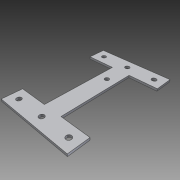
# Autodesk Inventor part: Shooter I Brace
Saved by Autodesk Inventor 2014 SP1 (Build 180222100, 222)
## iProperties
Created: 2013-12-15
Part Number: Shooter I Brace
Material: Aluminum 6061
Document SubType Name: Modeling
Designer: Moses
Mass: 64.49 g
Surface Area: 175.547 cm^2
Volume: 23.7971 cm^3
Density: 2.71 g/cm^3
Appearance: Aluminum - Flat
Author: Moses
Autodesk Inventor part; units mm, degrees
ref_plane "YZ Plane" through (0, 0, 0) normal (1, 0, 0) x (0, 1, 0)
ref_plane "XZ Plane" through (0, 0, 0) normal (0, 1, 0) x (-1, 0, 0)
ref_plane "XY Plane" through (0, 0, 0) normal (0, 0, 1) x (1, 0, 0)
sketch "Sketch1" plane through (0, 0, 0) normal (0, 1, 0) x (-1, 0, 0)
  line L0 (0, 0) -> (0, 25.4)
  line L1 (0, 0) -> (101.6, 0)
  line L2 (101.6, 0) -> (101.6, 25.4)
  line L3 (101.6, 25.4) -> (63.5, 25.4)
  line L4 (63.5, 25.4) -> (63.5, 127)
  line L5 (63.5, 127) -> (101.6, 127)
  line L6 (101.6, 127) -> (101.6, 152.4)
  line L7 (101.6, 152.4) -> (0, 152.4)
  line L8 (0, 152.4) -> (0, 127)
  line L9 (0, 127) -> (38.1, 127)
  line L10 (38.1, 127) -> (38.1, 25.4)
  line L11 (38.1, 25.4) -> (0, 25.4)
  line L12 (0, 139.7) -> (101.6, 139.7) construction
  line L13 (0, 12.7) -> (101.6, 12.7) construction
  line L14 (50.8, 0) -> (50.8, 152.4) construction
  circle A0 centre (12.7, 139.7) radius 3.3782
  circle A1 centre (50.8, 139.7) radius 3.3782
  circle A2 centre (12.7, 12.7) radius 3.3782
  circle A3 centre (50.8, 12.7) radius 3.3782
  circle A4 centre (88.9, 139.7) radius 3.3782
  circle A5 centre (88.9, 12.7) radius 3.3782
  circle A6 centre (50.8, 57.15) radius 3.3782
  circle A7 centre (50.8, 31.75) radius 3.3782
  circle A8 centre (50.8, 49.3713) radius 3.175 projected
  dimension "d0" = 25.4
  dimension "d1" = 101.6
  dimension "d4" = 38.1
  dimension "d5" = 6.7564
  dimension "d6" = 12.7
  dimension "d9" = 38.1
  dimension "d12" = 127
  dimension "d15" = 152.4
  dimension "d16" = 25.4
  dimension "d17" = 19.05
  dimension "d20" = 23.9713
  constraints: 30 end point, 8 centre point, 7 horizontal, 7 vertical, 6 equal length, 6 midpoint, 3 point on line, 2 equal radius, 10 other
  measures "d0" distance of L0.start L0.end
  measures "d1" distance of L0.start L1.end
  measures "d4" distance of L10.end L0.end
  measures "d5" diameter of A0
  measures "d6" distance from line of L8 A0.centre
  measures "d9" distance of A0.centre A1.centre
  measures "d12" distance of A0.centre A2.centre
  measures "d15" distance from line of L7 L0.start
  measures "d16" distance of A7.centre A6.centre
  measures "d17" distance of A3.centre A7.centre
  measures "d20" distance from line of L3 A8.centre
extrude "Extrusion1" add sketch "Sketch1" along normal blind 3.175 contours L0 L11 L10 L9 L8 L7 L6 L5 L4 L3 L2 L1 | A6 | A7
body "Solid1"
